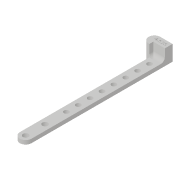
# Autodesk Inventor part: CollectorArmRear4_575long
Saved by Autodesk Inventor 2018 (Build 220112000, 112)
## iProperties
Created: 2019-02-19
Part Number: CollectorArmRear4_575long
Material: Generic
Document SubType Name: Modeling
Designer: ball
Density: 1 g/cm^3
Appearance: Default
Author: ball
Autodesk Inventor part; units mm, degrees
note: some values were not read from the file. Chosen so that the rebuilt part matches the saved one: direction of "Emboss1".
ref_plane "YZ Plane" through (0, 0, 0) normal (1, 0, 0) x (0, 1, 0)
ref_plane "XZ Plane" through (0, 0, 0) normal (0, 1, 0) x (-1, 0, 0)
ref_plane "XY Plane" through (0, 0, 0) normal (0, 0, 1) x (1, 0, 0)
sketch "Sketch1" plane through (0, 0, 0) normal (0, 1, 0) x (-1, 0, 0)
  line L0 (0, 0) -> (10.16, 0)
  line L1 (9.525, 9.6012) -> (9.525, 116.205)
  line L2 (0, 116.205) -> (0, 0)
  circle A0 centre (4.7625, 116.205) radius 2.2479
  circle A1 centre (4.7625, 100.203) radius 2.2479
  circle A2 centre (4.7625, 82.6516) radius 1.9685
  arc A3 (10.16, 0) -> (10.16, 9.6012) centre (10.16, 4.8006) ccw
  line L3 (10.16, 9.6012) -> (9.525, 9.6012)
  circle A4 centre (4.7625, 72.8726) radius 1.9685
  circle A5 centre (4.7625, 63.0936) radius 1.9685
  circle A6 centre (4.7625, 53.3146) radius 1.9685
  circle A7 centre (4.7625, 43.5356) radius 1.9685
  circle A8 centre (4.7625, 33.7566) radius 1.9685
  circle A9 centre (4.7625, 23.9776) radius 1.9685
  circle A10 centre (4.7625, 14.1986) radius 1.9685
  arc A11 (9.525, 116.205) -> (0, 116.205) centre (4.7625, 116.2555) ccw
  dimension "d0" = 9.525
  dimension "d4" = 4.4958
  dimension "d5" = 4.4958
  dimension "d6" = 16.002
  dimension "d7" = 3.937
  dimension "d8" = 17.5514
  dimension "d16" = 4.8006
  dimension "d17" = 10.16
  dimension "d18" = 116.205
  dimension "d21" = 9.779
  dimension "d27" = 4.7628
  dimension "d28" = 0
  dimension "d29" = 0
  constraints: 12 centre point, 8 end point, 4 point on circle, 2 perpendicular, 1 coincident, 1 horizontal, 1 parallel, 1 vertical, 14 other
  measures "d0" distance of L2.start L1.end
  measures "d4" diameter of A0
  measures "d5" diameter of A1
  measures "d6" distance of A1.centre A0.centre
  measures "d7" diameter of A2
  measures "d8" distance of A2.centre A1.centre
  measures "d16" distance from line of L0 point (10.16, 4.801)
  measures "d17" distance from line of L2 point (10.16, 4.801)
  measures "d18" distance from line of L0 A0.centre
  measures "d21" distance of A2.centre A4.centre
  measures "d27" radius of A11
  measures "d28" vertical distance of L1.end A0.centre
  measures "d29" vertical distance of L2.start A0.centre
extrude "Extrusion1" add sketch "Sketch1" along normal blind 3.175
sketch "Sketch2" plane through (0, 3.175, 0) normal (0, 1, 0) x (1, 0, 0)
  line L0 (-9.525, -9.6012) -> (-9.525, -6.35)
  line L1 (-9.525, -6.35) -> (0, -6.35)
  line L2 (0, -116.205) -> (0, 0) projected
  line L3 (0, -6.35) -> (0, 0)
  arc A0 (-10.16, 0) -> (-10.16, -9.6012) centre (-10.16, -4.8006) ccw projected
  arc A1 (-10.16, 0) -> (-10.239, -9.6012) centre (-10.1597, -4.8009) ccw
  line L4 (-10.16, -9.6012) -> (-9.525, -9.6012) projected
  line L5 (-9.525, -9.6012) -> (-10.16, -9.6012)
  line L6 (0, 0) -> (-10.16, 0) projected
  line L7 (-10.16, 0) -> (0, 0)
  constraints: 10 end point, 3 point on circle, 2 perpendicular, 1 centre point, 1 collinear, 1 horizontal, 1 vertical
extrude "Extrusion2" add sketch "Sketch2" along normal blind 9.525
fillet "Fillet1" radius 3.175 2 edges at (-4.7625, 3.175, 6.35) (-9.525, 3.175, 7.9756)
sketch "Sketch5" plane through (0, 12.7, 0) normal (0, 1, 0) x (1, 0, 0)
  line L0 (-11.1912, 0.0281) -> (-1.5184, 0.0281) construction
  line L1 (-1.5184, 0.0281) -> (-1.5184, -6.3829) construction
  line L2 (-1.5184, -6.3829) -> (-11.1912, -6.3829) construction
  line L3 (-11.1912, -6.3829) -> (-11.1912, 0.0281) construction
  line L4 (-9.1953, -3.8278) -> (-9.5391, -3.8278)
  line L5 (-9.5391, -3.8278) -> (-9.5391, -4.4268)
  line L6 (-9.5391, -4.4268) -> (-10.1545, -4.4268)
  line L7 (-10.1545, -4.4268) -> (-10.1545, -3.8278)
  line L8 (-10.1545, -3.8278) -> (-11.2742, -3.8278)
  line L9 (-11.2742, -3.8278) -> (-11.2742, -3.3544)
  line L10 (-11.2742, -3.3544) -> (-10.1751, -1.8806)
  line L11 (-10.1751, -1.8806) -> (-9.5391, -1.8806)
  line L12 (-9.5391, -1.8806) -> (-9.5391, -3.3709)
  line L13 (-9.5391, -3.3709) -> (-9.1953, -3.3709)
  line L14 (-9.1953, -3.3709) -> (-9.1953, -3.8278)
  line L15 (-10.1545, -3.3709) -> (-10.1545, -2.5064)
  line L16 (-10.1545, -2.5064) -> (-10.7988, -3.3709)
  line L17 (-10.7988, -3.3709) -> (-10.1545, -3.3709)
  line L18 (-8.2793, -4.4206) -> (-8.8824, -4.4206)
  line L19 (-8.8824, -4.4206) -> (-8.8824, -3.7496)
  line L20 (-8.8824, -3.7496) -> (-8.2793, -3.7496)
  line L21 (-8.2793, -3.7496) -> (-8.2793, -4.4206)
  spline S0 degree 2 poles (-5.9678, -3.5602) (-5.9678, -3.7599) (-6.1037, -4.0975) (-6.2375, -4.2189) knots 0 0 0 1 2 2 2
  spline S1 degree 2 poles (-6.2375, -4.2189) (-6.3713, -4.3404) (-6.7376, -4.4742) (-7.0052, -4.4742) knots 0 0 0 1 2 2 2
  spline S2 degree 2 poles (-7.0052, -4.4742) (-7.2893, -4.4721) (-7.6968, -4.3795) (-7.8306, -4.3198) knots 0 0 0 1 2 2 2
  line L22 (-7.8306, -4.3198) -> (-7.8306, -3.7661)
  line L23 (-7.8306, -3.7661) -> (-7.773, -3.7661)
  spline S3 degree 2 poles (-7.773, -3.7661) (-7.7236, -3.7928) (-7.6042, -3.8628) (-7.5075, -3.8999) knots 0 0 0 1 2 2 2
  spline S4 degree 2 poles (-7.5075, -3.8999) (-7.4169, -3.9349) (-7.2296, -3.9822) (-7.1164, -3.9822) knots 0 0 0 1 2 2 2
  spline S5 degree 2 poles (-7.1164, -3.9822) (-7.0176, -3.9822) (-6.787, -3.9328) (-6.7171, -3.8669) knots 0 0 0 1 2 2 2
  spline S6 degree 2 poles (-6.7171, -3.8669) (-6.6656, -3.8155) (-6.608, -3.6899) (-6.608, -3.5849) knots 0 0 0 1 2 2 2
  spline S7 degree 2 poles (-6.608, -3.5849) (-6.608, -3.4944) (-6.6821, -3.3668) (-6.7418, -3.3277) knots 0 0 0 1 2 2 2
  spline S8 degree 2 poles (-6.7418, -3.3277) (-6.8282, -3.27) (-7.0752, -3.2371) (-7.1637, -3.2371) knots 0 0 0 1 2 2 2
  spline S9 degree 2 poles (-7.1637, -3.2371) (-7.3037, -3.2371) (-7.5692, -3.2824) (-7.666, -3.3071) knots 0 0 0 1 2 2 2
  line L24 (-7.666, -3.3071) -> (-7.7215, -3.3071)
  line L25 (-7.7215, -3.3071) -> (-7.7215, -1.8806)
  line L26 (-7.7215, -1.8806) -> (-6.0378, -1.8806)
  line L27 (-6.0378, -1.8806) -> (-6.0378, -2.3602)
  line L28 (-6.0378, -2.3602) -> (-7.1184, -2.3602)
  line L29 (-7.1184, -2.3602) -> (-7.1184, -2.7822)
  spline S10 degree 2 poles (-7.1184, -2.7822) (-7.067, -2.7781) (-6.925, -2.774) (-6.8858, -2.774) knots 0 0 0 1 2 2 2
  spline S11 degree 2 poles (-6.8858, -2.774) (-6.7027, -2.774) (-6.3939, -2.8481) (-6.2725, -2.9242) knots 0 0 0 1 2 2 2
  spline S12 degree 2 poles (-6.2725, -2.9242) (-6.1284, -3.0189) (-5.9678, -3.3338) (-5.9678, -3.5602) knots 0 0 0 1 2 2 2
  line L30 (-3.7407, -2.3849) -> (-4.8254, -4.4206)
  line L31 (-4.8254, -4.4206) -> (-5.5335, -4.4206)
  line L32 (-5.5335, -4.4206) -> (-4.3994, -2.3602)
  line L33 (-4.3994, -2.3602) -> (-5.6097, -2.3602)
  line L34 (-5.6097, -2.3602) -> (-5.6097, -1.8806)
  line L35 (-5.6097, -1.8806) -> (-3.7407, -1.8806)
  line L36 (-3.7407, -1.8806) -> (-3.7407, -2.3849)
  spline S13 degree 2 poles (-1.5177, -3.5602) (-1.5177, -3.7599) (-1.6535, -4.0975) (-1.7873, -4.2189) knots 0 0 0 1 2 2 2
  spline S14 degree 2 poles (-1.7873, -4.2189) (-1.9211, -4.3404) (-2.2875, -4.4742) (-2.5551, -4.4742) knots 0 0 0 1 2 2 2
  spline S15 degree 2 poles (-2.5551, -4.4742) (-2.8391, -4.4721) (-3.2467, -4.3795) (-3.3805, -4.3198) knots 0 0 0 1 2 2 2
  line L37 (-3.3805, -4.3198) -> (-3.3805, -3.7661)
  line L38 (-3.3805, -3.7661) -> (-3.3228, -3.7661)
  spline S16 degree 2 poles (-3.3228, -3.7661) (-3.2734, -3.7928) (-3.1541, -3.8628) (-3.0573, -3.8999) knots 0 0 0 1 2 2 2
  spline S17 degree 2 poles (-3.0573, -3.8999) (-2.9668, -3.9349) (-2.7794, -3.9822) (-2.6662, -3.9822) knots 0 0 0 1 2 2 2
  spline S18 degree 2 poles (-2.6662, -3.9822) (-2.5674, -3.9822) (-2.3369, -3.9328) (-2.2669, -3.8669) knots 0 0 0 1 2 2 2
  spline S19 degree 2 poles (-2.2669, -3.8669) (-2.2155, -3.8155) (-2.1578, -3.6899) (-2.1578, -3.5849) knots 0 0 0 1 2 2 2
  spline S20 degree 2 poles (-2.1578, -3.5849) (-2.1578, -3.4944) (-2.2319, -3.3668) (-2.2916, -3.3277) knots 0 0 0 1 2 2 2
  spline S21 degree 2 poles (-2.2916, -3.3277) (-2.3781, -3.27) (-2.6251, -3.2371) (-2.7136, -3.2371) knots 0 0 0 1 2 2 2
  spline S22 degree 2 poles (-2.7136, -3.2371) (-2.8535, -3.2371) (-3.1191, -3.2824) (-3.2158, -3.3071) knots 0 0 0 1 2 2 2
  line L39 (-3.2158, -3.3071) -> (-3.2714, -3.3071)
  line L40 (-3.2714, -3.3071) -> (-3.2714, -1.8806)
  line L41 (-3.2714, -1.8806) -> (-1.5877, -1.8806)
  line L42 (-1.5877, -1.8806) -> (-1.5877, -2.3602)
  line L43 (-1.5877, -2.3602) -> (-2.6683, -2.3602)
  line L44 (-2.6683, -2.3602) -> (-2.6683, -2.7822)
  spline S23 degree 2 poles (-2.6683, -2.7822) (-2.6168, -2.7781) (-2.4748, -2.774) (-2.4357, -2.774) knots 0 0 0 1 2 2 2
  spline S24 degree 2 poles (-2.4357, -2.774) (-2.2525, -2.774) (-1.9438, -2.8481) (-1.8223, -2.9242) knots 0 0 0 1 2 2 2
  spline S25 degree 2 poles (-1.8223, -2.9242) (-1.6782, -3.0189) (-1.5177, -3.3338) (-1.5177, -3.5602) knots 0 0 0 1 2 2 2
  point P0 (0, 0)
  constraints: 2 other
emboss "Emboss1" sketch "Sketch5" operation cut depth 0.762 direction (0, -1, 0)
body "Solid1"
